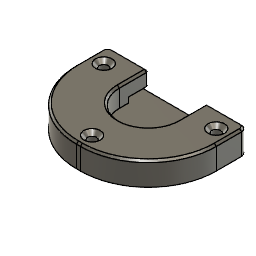
filamentspoolholder (Autodesk Fusion 360 design; units mm, degrees)
Autodesk Fusion 360 part; units mm, degrees
sketch "Sketch1" plane through (0, 0, 0) normal (0, 1, 0) x (1, 0, 0)
  circle A0 centre (0, 0) radius 15
  line L0 (-15, 0) -> (-15, 15)
  line L1 (-15, 15) -> (15, 15)
  line L2 (15, 15) -> (15, 0)
  line L3 (-15, 15) -> (-18.075, 15)
  line L4 (-18.075, 15) -> (-18.075, 4.85)
  line L5 (-18.075, 4.85) -> (-15, 4.85)
  line L6 (15, 15) -> (18.075, 15)
  line L7 (18.075, 15) -> (18.075, 4.85)
  line L8 (18.075, 4.85) -> (14.975, 4.85)
  line L9 (-7.875, -16.2971) -> (-7.875, -12.7665)
  line L10 (7.875, -16.2971) -> (7.875, -12.7665)
  line L11 (-7.875, -12.7665) -> (-7.875, -16.2971)
  line L12 (7.875, -12.7665) -> (7.875, -16.2971)
  arc A1 (-7.875, -16.2971) -> (7.875, -16.2971) centre (0, 0) ccw
  circle A2 centre (0, 0) radius 22
  line L13 (-22, 0) -> (-22, 22)
  line L14 (-22, 22) -> (22, 22)
  line L15 (22, 22) -> (22, 0)
  line L16 (-18.075, 15) -> (-22, 15)
  line L17 (18.075, 15) -> (22, 15)
  point P0 (0, -18.1)
  dimension "d1" = 30
  dimension "d3" = 10.15
  dimension "d5" = 15.75
  dimension "d6" = 36.15
  dimension "d7" = 18.1
  dimension "d8" = 7
  dimension "d9" = -7
  constraint coincident A0.centre A1.centre
  constraint coincident A0 L0.start
  constraint tangent A0 L0
  constraint vertical L0
  constraint perpendicular L0 L1
  constraint coincident A0 L2.end
  constraint tangent A0 L2
  constraint tangent A0 L1
  constraint perpendicular L1 L2
  constraint perpendicular L0 L3
  constraint perpendicular L3 L4
  constraint coincident L0 L5.end
  constraint perpendicular L0 L5
  constraint perpendicular L2 L6
  constraint perpendicular L6 L7
  constraint perpendicular L2 L8
  constraint equal L3 L6
  constraint equal L4 L7
  constraint coincident A0 L9.end
  constraint parallel L7 L9
  constraint coincident A0 L10.end
  constraint parallel L9 L10
  constraint equal L9 L10
  constraint midpoint A1 P0
  constraint coincident L13 L16.end
  constraint perpendicular L13 L16
  constraint coincident L15 L17.end
  constraint perpendicular L15 L17
  measures "d1" diameter of A0
  measures "d3" distance of L3.end L4.end
  measures "d5" distance of L9 L10
  measures "d6" distance of L4 L7
  measures "d7" distance of A0.centre P0
extrude "Extrude1" add sketch "Sketch1" along normal blind 12 contours A0 L0 L2 L4 L5 L7 L8 L9 L10 L11 L12 A1 A2 | A0 L9 L10 L11 L12 A1 | L0 L3 L4 L5 A2 | L2 L6 L7 L8 A2 | L3 L4 A2 | L6 L7 A2 | L4 A2 L13 L16 | L7 A2 L15 L17
extrude "Extrude2" add sketch "Sketch1" along normal blind 2 contours A0 | A0 L0 L1 | A0 L1 L2
extrude "Extrude3" cut sketch "Sketch1" along normal blind 2.7 from surface at 2 contours A0 L9 L10 L11 L12 A1 | L0 L3 L4 L5 A2 | L2 L6 L7 L8 A2 | L3 L4 A2 | L6 L7 A2
sketch "Sketch2" plane through (0, 0, 0) normal (0, 1, 0) x (1, 0, 0)
  line L0 (-36, 15) -> (36, 15)
  line L1 (36, 15) -> (36, -36)
  line L2 (36, -36) -> (-36, -36)
  line L3 (-36, -36) -> (-36, 15)
  line L4 (-22, 15) -> (-22, 0)
  arc A0 (-22, 0) -> (22, 0) centre (0, 0) ccw
  line L5 (-15, 15) -> (-22, 15)
  circle A1 centre (-29, 6) radius 2.25
  circle A2 centre (29, 6) radius 2.25
  circle A3 centre (0, -29) radius 2.25
  line L6 (0, -22) -> (0, -36) construction
  line L7 (-22, 15) -> (-36, 15) construction
  line L8 (36, 15) -> (22, 15) construction
  line L9 (22, 15) -> (22, 0)
  point P0 (0, -36)
  point P1 (0, -22)
  point P2 (0, -29)
  point P3 (22, 15)
  point P4 (-29, 15)
  point P5 (29, 15)
  dimension "d17" = 14
  dimension "d18" = 14
  dimension "d19" = 9
  dimension "d20" = 4.5
  constraint horizontal L0
  constraint vertical L1
  constraint horizontal L2
  constraint vertical L3
  constraint midpoint L2 P0
  constraint vertical A0.centre L6.end
  constraint vertical A0.centre P1
  constraint coincident P1 A0
  constraint collinear L0 L5
  constraint equal A1 A3
  constraint equal A2 A3
  constraint vertical P1 P2
  constraint coincident P1 L6.start
  constraint coincident P0 L6.end
  constraint midpoint L6 P2
  constraint coincident P2 A3.centre
  constraint coincident L4.start L5.end
  constraint coincident L0 P3
  constraint coincident P3 L8.end
  constraint midpoint L7 P4
  constraint vertical A1.centre P4
  constraint midpoint L8 P5
  constraint vertical A2.centre P5
  constraint horizontal A1.centre A2.centre
  measures "d17" distance of L3 L4
  measures "d18" distance of P0 P1
  measures "d19" distance of A2.centre P5
  measures "d20" diameter of A1
extrude "Extrude4" add sketch "Sketch2" along normal up to surface (12 mm away) contours L0 L1 L2 L3 L4 A0 L9
chamfer "Chamfer1" distance 2 angle 45 3 edges at (-31.0977, 12, -5.1864) (26.9023, 12, -5.1864) (-2.0977, 12, 29.8136)
fillet "Fillet1" radius 35 2 edges at (-36, 6, 36) (36, 6, 36)
fillet "Fillet2" radius 3 2 edges at (36, 6, -15) (-36, 6, -15)
fillet "Fillet3" radius 1 4 edges at (-15, 8.35, -15) (15, 8.35, -15) (-7.875, 3.35, 12.7665) (7.875, 3.35, 12.7665)
chamfer "Chamfer2" distance 1 angle 45 14 edges at (-25.7487, 12, 25.7487) (-36, 12, -5.5) (-35.1213, 12, -14.1213) (-24.5, 12, -15) (-15.2929, 12, -14.7071) (-15, 12, -7) (0, 12, 15) (15, 12, -7) (15.2929, 12, -14.7071) (24.5, 12, -15) (35.1213, 12, -14.1213) (36, 12, -5.5) (25.7487, 12, 25.7487) (0, 12, 36)
equation "d7 = d1 / 2 + 3.1 mm"
equation "d15 = 2.5 mm + 0.2 mm"
equation "d18 = d17"
